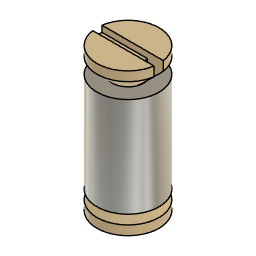
Tubo de estanho v1 (Autodesk Fusion 360 design; units mm, degrees)
Autodesk Fusion 360 part; units mm, degrees
note: some values were not read from the file. Set by a fixed rule: which sketch regions a step uses.
sketch "Sketch1" plane through (0, 0, 0) normal (0, 1, 0) x (1, 0, 0)
  line L0 (0, -46) -> (0, 0)
  line L1 (0, 0) -> (10, 0)
  line L2 (10, 0) -> (10, -3)
  line L3 (10, -3) -> (5, -8)
  line L4 (5, -8) -> (5, -38)
  line L5 (5, -38) -> (10, -43)
  line L6 (10, -43) -> (10, -46)
  line L7 (10, -46) -> (0, -46)
  dimension "d1" = 135
  dimension "d2" = 3
  dimension "d3" = 5
  dimension "d4" = 10
  dimension "d5" = 30
  constraint coincident L0.end L1.start
  constraint vertical L0
  constraint perpendicular L0 L1
  constraint perpendicular L1 L2
  constraint perpendicular L1 L4
  constraint parallel L4 L6
  constraint perpendicular L4 L7
  constraint equal L2 L6
  constraint equal L3 L5
  constraint equal L1 L7
  measures "d1" angle of L3 L4
  measures "d2" distance of L5.end L6.end
  measures "d3" distance of L0 L4
  measures "d4" distance of L6.end L0.start
  measures "d5" distance of L3.end L4.end
revolve "Revolve1" add sketch "Sketch1" angle 360 about axis through (0, 0, 46) along (0, 0, -1) makes body 1
sketch "Sketch2" plane through (0, 0, 46) normal (0, 0, 1) x (-1, 0, 0)
  circle A0 centre (0, 0) radius 10
  line L0 (9.8869, -1.5) -> (-9.8869, -1.5)
  line L1 (-9.8869, 1.5) -> (9.8869, 1.5)
  circle A1 centre (0, 0) radius 5 construction
  circle A2 centre (0, 0) radius 5
  line L2 (-4.7697, -1.5) -> (-4.7697, 1.5)
  dimension "d7" = 3
  constraint coincident A0 L0.start
  constraint coincident A0 L0.end
  constraint horizontal L0
  constraint coincident A0 L1.start
  constraint coincident A0 L1.end
  constraint parallel L0 L1
  constraint equal L0 L1
  constraint coincident A1 L2.start
  constraint coincident L0 L2.start
  constraint coincident A1 L2.end
  constraint coincident L1 L2.end
  measures "d7" distance of L0 L1
extrude "Extrude1" cut sketch "Sketch2" against normal blind 2 contours A0 L0 L1 A2 | L0 L1 A2 L2 | A2 L2 picked at (6.6539, -0.3362) bodies 1
extrude "Extrude2" cut sketch "Sketch2" against normal blind 16 contours A0 L0 L1 A2 picked at (-8.2883, -0.7687) bodies 1
extrude "Extrude3" add sketch "Sketch2" against normal blind 32 from surface at -8 separate body contours A0 L0 L1 A2 | A0 L1 A2 | A0 L0 A2 | A0 L0 L1 A2 | L0 L1 A2 L2 | L1 A2 | L0 A2 makes body 2
